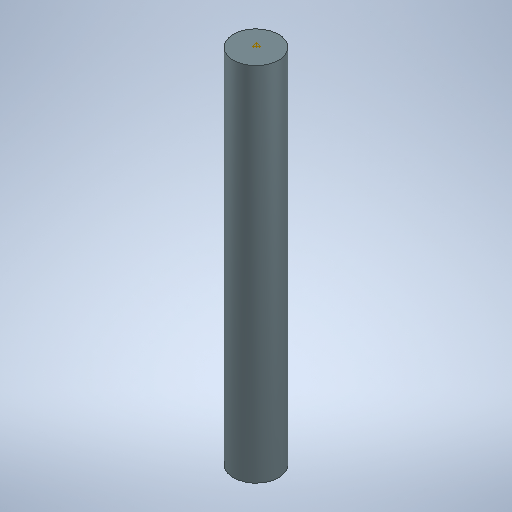
# Autodesk Inventor part: Heater
Saved by Autodesk Inventor 2025.3 (Build 293356000, 356)
## iProperties
Created: 2025-05-16
Part Number: Heater
Material: Generic
Document SubType Name: Modeling
Designer: Verðandi
Density: 1 g/cm^3
Appearance: Lead
Categories: <MemberInstance><Categories><Category DisplayName="" Mnemonic="CABLEANDHARNESS" InternalName="e4a7e005-5e42-4d16-b293-125e7f0d0512"><Category DisplayName="" Mnemonic="CONNECTORS" InternalName="6f634eba-a678-4820-a31d-2c2d5ee6728e"><CategoryParameter DisplayName="" Mnemonic="REFDES" InternalName="c3740e8c-60ab-4d5d-8584-52b73222f2f0"/><Category DisplayName="" Mnemonic="DISCRETEWIRE" InternalName="9a3407de-09b2-4cdb-8c40-9708d5144a28"/></Category></Category></Categories><FamilyTemplate><FamilyTemplateParameters></FamilyTemplateParameters></FamilyTemplate><CategoryParameterMap><ParamToTemplateMap><ParamToTemplate CategoryParameter="//CategoryParameter[@InternalName='c3740e8c-60ab-4d5d-8584-52b73222f2f0']" ConstantValue=""/></ParamToTemplateMap></CategoryParameterMap></MemberInstance>
Author: Verðandi
Autodesk Inventor part; units mm, degrees
ref_plane "YZ Plane" through (0, 0, 0) normal (1, 0, 0) x (0, 1, 0)
ref_plane "XZ Plane" through (0, 0, 0) normal (0, 1, 0) x (-1, 0, 0)
ref_plane "XY Plane" through (0, 0, 0) normal (0, 0, 1) x (1, 0, 0)
sketch "Sketch1" plane through (0, 0, 0) normal (0, 1, 0) x (-1, 0, 0)
  circle A0 centre (0, 0) radius 1.5875
  dimension "d0" = 3.175
  constraints: 1 centre point, 1 coincident
  measures "d0" diameter of A0
extrude "Extrusion1" add sketch "Sketch1" along normal blind 25.4
sketch "Sketch2" plane through (0, 25.4, 0) normal (0, 1, 0) x (1, 0, 0)
  circle A0 centre (0, 0) radius 1.5875 projected
body "Solid1"
